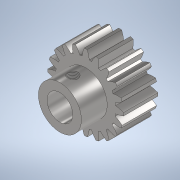
# Autodesk Inventor part: Spur Gear1
Saved by Autodesk Inventor 2020 (Build 240168000, 168)
## iProperties
CustomPartVersion: 1
Created: 2020-05-17
Part Number: Spur Gear1
Material: Steel, Mild
Document SubType Name: Modeling
Designer: Hesekiel
Categories: <?xml version="1.0" encoding="UTF-16"?> <MemberInstance><Categories><FamilyTemplate><FamilyTemplateParameter ValueType="xs:double" Id="1" ObjectReferenceKey="da_z" ObjectType="kUserParameterObject"/><FamilyTemplateParameter ValueType="xs:double" Id="2" ObjectReferenceKey="da_b" ObjectType="kUserParameterObject"/><FamilyTemplateParameter ValueType="xs:double" Id="3" ObjectReferenceKey="da_beta" ObjectType="kUserParameterObject"/><FamilyTemplateParameter ValueType="xs:double" Id="4" ObjectReferenceKey="da_da" ObjectType="kUserParameterObject"/><FamilyTemplateParameter ValueType="xs:double" Id="5" ObjectReferenceKey="da_aw" ObjectType="kUserParameterObject"/><FamilyTemplateParameter ValueType="xs:string" Id="6" ObjectReferenceKey="EAIAABAAAACIAQAAAAAAAIAAAAAAAAAA" ObjectType="83910656" SubObjectId="SurfaceGeometry"/></FamilyTemplate><ParamToTemplateMap><ParamToTemplate CategoryParameter="//CategoryParameter[@InternalName='046C89C9-8512-4d59-83FE-43B91F4F132A']" TemplateParameter="1"/><ParamToTemplate CategoryParameter="//CategoryParameter[@InternalName='2552DF32-E462-4b46-AEBF-C6C7768E72AC']" TemplateParameter="2"/><ParamToTemplate CategoryParameter="//CategoryParameter[@InternalName='C9EE641D-15FC-4fae-A226-E94C4372FDD7']" TemplateParameter="3"/><ParamToTemplate><ParamToTemplate CategoryParameter="//CategoryParameter[@InternalName='00B6519A-459B-49c7-AD84-2E56D39A5744']" ConstantValue="0.000000"/></ParamToTemplate><ParamToTemplate><ParamToTemplate CategoryParameter="//CategoryParameter[@InternalName='04B31F0E-C7A6-4894-AA32-9629BEFACF47']" ConstantValue="1.000000"/></ParamToTemplate><ParamToTemplate><ParamToTemplate CategoryParameter="//CategoryParameter[@InternalName='43CBEC2E-7847-49e7-A936-2F7889FCB2D9']" ConstantValue="0.250000"/></ParamToTemplate><ParamToTemplate><ParamToTemplate CategoryParameter="//CategoryParameter[@InternalName='B1EFC894-105D-4ebd-86BF-FA20ED196853']" ConstantValue="0.350000"/></ParamToTemplate><ParamToTemplate><ParamToTemplate CategoryParameter="//CategoryParameter[@InternalName='51175063-3D10-4879-93E8-6246FE8B403D']" ConstantValue="2060000000.000000"/></ParamToTemplate><ParamToTemplate><ParamToTemplate CategoryParameter="//CategoryParameter[@InternalName='A3A52E27-4454-46a9-B0BD-C932399B70AF']" ConstantValue="0.300000"/></ParamToTemplate><ParamToTemplate><ParamToTemplate CategoryParameter="//CategoryParameter[@InternalName='91B76062-C214-41d9-B1B9-14D2AB99603D']" ConstantValue="0.200000"/></ParamToTemplate><ParamToTemplate><ParamToTemplate CategoryParameter="//CategoryParameter[@InternalName='374E806E-8B8A-4dda-A9AA-1039D6500AD2']" ConstantValue="5.000000"/></ParamToTemplate><ParamToTemplate><ParamToTemplate CategoryParameter="//CategoryParameter[@InternalName='2D373A89-B862-43d6-8D0B-0CBF12AB9F6C']" ConstantValue="0.349066"/></ParamToTemplate><ParamToTemplate CategoryParameter="//CategoryParameter[@InternalName='37777632-D6A2-4fac-9D53-DB8ACD95C989']" TemplateParameter="4"/><ParamToTemplate CategoryParameter="//CategoryParameter[@InternalName='FD1017F1-B727-4f7e-9707-0F86F1FF9423']" TemplateParameter="5"/><ParamToTemplate><ParamToTemplate CategoryParameter="//CategoryParameter[@InternalName='9E1B4470-B2D3-4ff1-B813-535BB4CDF51A']" ConstantValue="3520000.000000"/></ParamToTemplate><ParamToTemplate><ParamToTemplate CategoryParameter="//CategoryParameter[@InternalName='F8452263-BFF6-458c-9FB1-07C4B99E95CD']" ConstantValue="11400000.000000"/></ParamToTemplate><ParamToTemplate><ParamToTemplate CategoryParameter="//CategoryParameter[@InternalName='3E3BB259-FD49-497f-8171-6EBC954A3479']" ConstantValue="2.000000"/></ParamToTemplate><ParamToTemplate CategoryParameter="//CategoryParameter[@InternalName='27C3BAF2-7550-4e4b-AE2C-0DB134B7D9B7']" TemplateParameter="6"/></ParamToTemplateMap><Category DisplayName="Gear" InternalName="DC85795E-93AB-48d5-8EEE-5A27447B64BD" Mnemonic="Gear"><CategoryParameter DisplayName="z" InternalName="046C89C9-8512-4d59-83FE-43B91F4F132A" Mnemonic="z"/><CategoryParameter DisplayName="b" InternalName="2552DF32-E462-4b46-AEBF-C6C7768E72AC" Mnemonic="b"/><CategoryParameter DisplayName="||b|" InternalName="C9EE641D-15FC-4fae-A226-E94C4372FDD7" Mnemonic="beta"/><CategoryParameter DisplayName="x" InternalName="00B6519A-459B-49c7-AD84-2E56D39A5744" Mnemonic="x"/><CategoryParameter DisplayName="a*" InternalName="04B31F0E-C7A6-4894-AA32-9629BEFACF47" Mnemonic="a"/><CategoryParameter DisplayName="c*" InternalName="43CBEC2E-7847-49e7-A936-2F7889FCB2D9" Mnemonic="c"/><CategoryParameter DisplayName="r|.f|*" InternalName="B1EFC894-105D-4ebd-86BF-FA20ED196853" Mnemonic="rf"/><CategoryParameter DisplayName="E" InternalName="51175063-3D10-4879-93E8-6246FE8B403D" Mnemonic="E"/><CategoryParameter DisplayName="||m|" InternalName="A3A52E27-4454-46a9-B0BD-C932399B70AF" Mnemonic="mi"/><Category DisplayName="SpurGear" InternalName="26C5A22E-A91E-4dfd-A3B3-23CCAFAE1764" Mnemonic="SpurGear"><CategoryParameter DisplayName="m" InternalName="91B76062-C214-41d9-B1B9-14D2AB99603D" Mnemonic="m"/><CategoryParameter DisplayName="P" InternalName="374E806E-8B8A-4dda-A9AA-1039D6500AD2" Mnemonic="PP"/><CategoryParameter DisplayName="||a|" InternalName="2D373A89-B862-43d6-8D0B-0CBF12AB9F6C" Mnemonic="alpha"/><CategoryParameter DisplayName="d|.a|" InternalName="37777632-D6A2-4fac-9D53-DB8ACD95C989" Mnemonic="da"/><CategoryParameter DisplayName="a|.w|" InternalName="FD1017F1-B727-4f7e-9707-0F86F1FF9423" Mnemonic="aw"/><CategoryParameter DisplayName="||s||.Flim|" InternalName="9E1B4470-B2D3-4ff1-B813-535BB4CDF51A" Mnemonic="sFlim"/><CategoryParameter DisplayName="||s||.Hlim|" InternalName="F8452263-BFF6-458c-9FB1-07C4B99E95CD" Mnemonic="sHlim"/><CategoryParameter DisplayName="type" InternalName="3E3BB259-FD49-497f-8171-6EBC954A3479" Mnemonic="type"/><CategoryParameter DisplayName="PitchDiameter" InternalName="27C3BAF2-7550-4e4b-AE2C-0DB134B7D9B7" Mnemonic="IDS_PITCHDIAM"/></Category></Category></Categories></MemberInstance>
Density: 7.85 g/cm^3
Appearance: Semi-Polished
Mass: 203.835 g
Surface Area: 100.654 cm^2
Volume: 25.9662 cm^3
Author: Hesekiel
Autodesk Inventor part; units mm, degrees
sketch "Sketch1" plane through (0, 0, 0) normal (0, 0, 1) x (1, 0, 0)
  circle A0 centre (0, 0) radius 22
  dimension "d0" = 44
  constraints: 1 centre point
  measures "d0" diameter of A0
extrude "Extrusion1" add sketch "Sketch1" along normal blind 20
ref_plane "Work Plane2" through (0, 0, 10) normal (0, 0, 1) x (1, 0, 0)
sketch "Sketch2" plane through (0, 0, 0) normal (0, 0, -1) x (-1, 0, 0)
  circle A0 centre (0, 0) radius 22 projected
  circle A1 centre (0, 0) radius 20
  dimension "d3" = 40
  constraints: 1 centre point, 1 coincident
  measures "d3" diameter of A1
surface extrude "Pitch Diameter" sketch "Sketch2" against normal through all shown no curves A1
ref_plane "Work Plane8" through (0, 0, 0) normal (0.9876883, 0.1564345, 0) x (0, 0, 1)
ref_plane "Work Plane9" through (0, 0, 0) normal (1, 0, 0) x (0, 1, 0)
spur gear teeth "Spur Gear" teeth 20 pitch diameter 40 tip diameter 44 root diameter 35 face width 20 start plane through (0, 0, 0) normal (0, 0, -1) x (-1, 0, 0)
sketch "Sketch3" plane through (0, 0, 20) normal (0, 0, 1) x (1, 0, 0)
  circle A0 centre (0, 0) radius 7.5
  dimension "d49" = 15
  constraints: 1 centre point, 1 coincident
  measures "d49" diameter of A0
extrude "Extrusion2" cut sketch "Sketch3" against normal up to surface (20 mm away)
sketch "Sketch4" plane through (0, 0, 20) normal (0, 0, 1) x (1, 0, 0)
  circle A0 centre (0, 0) radius 12.5
  circle A1 centre (0, 0) radius 7.5 projected
  arc A2 (-7.6146, 20.6402) -> (-7.3265, 15.8925) centre (8.9064, 19.2599) ccw projected
  arc A3 (-7.3265, 15.8925) -> (-8.5509, 15.2687) centre (0, 0) ccw projected
  arc A4 (-8.5509, 15.2687) -> (-12.2225, 18.2923) centre (-20.8166, 4.1153) ccw projected
  arc A5 (-12.2225, 18.2923) -> (-13.6201, 17.277) centre (0, 0) ccw projected
  arc A6 (-13.6201, 17.277) -> (-11.879, 12.8506) centre (2.5188, 21.0695) ccw projected
  arc A7 (-11.879, 12.8506) -> (-12.8506, 11.879) centre (0, 0) ccw projected
  arc A8 (-12.8506, 11.879) -> (-17.277, 13.6201) centre (-21.0695, -2.5188) ccw projected
  arc A9 (-17.277, 13.6201) -> (-18.2923, 12.2225) centre (0, 0) ccw projected
  arc A10 (-18.2923, 12.2225) -> (-15.2687, 8.5509) centre (-4.1153, 20.8166) ccw projected
  arc A11 (-15.2687, 8.5509) -> (-15.8925, 7.3265) centre (0, 0) ccw projected
  arc A12 (-15.8925, 7.3265) -> (-20.6402, 7.6146) centre (-19.2599, -8.9064) ccw projected
  arc A13 (-20.6402, 7.6146) -> (-21.174, 5.9717) centre (0, 0) ccw projected
  arc A14 (-21.174, 5.9717) -> (-17.1637, 3.4141) centre (-10.3466, 18.5261) ccw projected
  arc A15 (-17.1637, 3.4141) -> (-17.3787, 2.0569) centre (0, 0) ccw projected
  arc A16 (-17.3787, 2.0569) -> (-21.983, 0.8637) centre (-15.565, -14.4221) ccw projected
  arc A17 (-21.983, 0.8637) -> (-21.983, -0.8637) centre (0, 0) ccw projected
  arc A18 (-21.983, -0.8637) -> (-17.3787, -2.0569) centre (-15.565, 14.4221) ccw projected
  arc A19 (-17.3787, -2.0569) -> (-17.1637, -3.4141) centre (0, 0) ccw projected
  arc A20 (-17.1637, -3.4141) -> (-21.174, -5.9717) centre (-10.3466, -18.5261) ccw projected
  arc A21 (-21.174, -5.9717) -> (-20.6402, -7.6146) centre (0, 0) ccw projected
  arc A22 (-20.6402, -7.6146) -> (-15.8925, -7.3265) centre (-19.2599, 8.9064) ccw projected
  arc A23 (-15.8925, -7.3265) -> (-15.2687, -8.5509) centre (0, 0) ccw projected
  arc A24 (-15.2687, -8.5509) -> (-18.2923, -12.2225) centre (-4.1153, -20.8166) ccw projected
  arc A25 (-18.2923, -12.2225) -> (-17.277, -13.6201) centre (0, 0) ccw projected
  arc A26 (-17.277, -13.6201) -> (-12.8506, -11.879) centre (-21.0695, 2.5188) ccw projected
  arc A27 (-12.8506, -11.879) -> (-11.879, -12.8506) centre (0, 0) ccw projected
  arc A28 (-11.879, -12.8506) -> (-13.6201, -17.277) centre (2.5188, -21.0695) ccw projected
  arc A29 (-13.6201, -17.277) -> (-12.2225, -18.2923) centre (0, 0) ccw projected
  arc A30 (-12.2225, -18.2923) -> (-8.5509, -15.2687) centre (-20.8166, -4.1153) ccw projected
  arc A31 (-8.5509, -15.2687) -> (-7.3265, -15.8925) centre (0, 0) ccw projected
  arc A32 (-7.3265, -15.8925) -> (-7.6146, -20.6402) centre (8.9064, -19.2599) ccw projected
  arc A33 (-7.6146, -20.6402) -> (-5.9717, -21.174) centre (0, 0) ccw projected
  arc A34 (-5.9717, -21.174) -> (-3.4141, -17.1637) centre (-18.5261, -10.3466) ccw projected
  arc A35 (-3.4141, -17.1637) -> (-2.0569, -17.3787) centre (0, 0) ccw projected
  arc A36 (-2.0569, -17.3787) -> (-0.8637, -21.983) centre (14.4221, -15.565) ccw projected
  arc A37 (-0.8637, -21.983) -> (0.8637, -21.983) centre (0, 0) ccw projected
  arc A38 (0.8637, -21.983) -> (2.0569, -17.3787) centre (-14.4221, -15.565) ccw projected
  arc A39 (2.0569, -17.3787) -> (3.4141, -17.1637) centre (0, 0) ccw projected
  arc A40 (3.4141, -17.1637) -> (5.9717, -21.174) centre (18.5261, -10.3466) ccw projected
  arc A41 (5.9717, -21.174) -> (7.6146, -20.6402) centre (0, 0) ccw projected
  arc A42 (7.6146, -20.6402) -> (7.3265, -15.8925) centre (-8.9064, -19.2599) ccw projected
  arc A43 (7.3265, -15.8925) -> (8.5509, -15.2687) centre (0, 0) ccw projected
  arc A44 (8.5509, -15.2687) -> (12.2225, -18.2923) centre (20.8166, -4.1153) ccw projected
  arc A45 (12.2225, -18.2923) -> (13.6201, -17.277) centre (0, 0) ccw projected
  arc A46 (13.6201, -17.277) -> (11.879, -12.8506) centre (-2.5188, -21.0695) ccw projected
  arc A47 (11.879, -12.8506) -> (12.8506, -11.879) centre (0, 0) ccw projected
  arc A48 (12.8506, -11.879) -> (17.277, -13.6201) centre (21.0695, 2.5188) ccw projected
  arc A49 (17.277, -13.6201) -> (18.2923, -12.2225) centre (0, 0) ccw projected
  arc A50 (18.2923, -12.2225) -> (15.2687, -8.5509) centre (4.1153, -20.8166) ccw projected
  arc A51 (15.2687, -8.5509) -> (15.8925, -7.3265) centre (0, 0) ccw projected
  arc A52 (15.8925, -7.3265) -> (20.6402, -7.6146) centre (19.2599, 8.9064) ccw projected
  arc A53 (20.6402, -7.6146) -> (21.174, -5.9717) centre (0, 0) ccw projected
  arc A54 (21.174, -5.9717) -> (17.1637, -3.4141) centre (10.3466, -18.5261) ccw projected
  arc A55 (17.1637, -3.4141) -> (17.3787, -2.0569) centre (0, 0) ccw projected
  arc A56 (17.3787, -2.0569) -> (21.983, -0.8637) centre (15.565, 14.4221) ccw projected
  arc A57 (21.983, -0.8637) -> (21.983, 0.8637) centre (0, 0) ccw projected
  arc A58 (21.983, 0.8637) -> (17.3787, 2.0569) centre (15.565, -14.4221) ccw projected
  arc A59 (17.3787, 2.0569) -> (17.1637, 3.4141) centre (0, 0) ccw projected
  arc A60 (17.1637, 3.4141) -> (21.174, 5.9717) centre (10.3466, 18.5261) ccw projected
  arc A61 (21.174, 5.9717) -> (20.6402, 7.6146) centre (0, 0) ccw projected
  arc A62 (20.6402, 7.6146) -> (15.8925, 7.3265) centre (19.2599, -8.9064) ccw projected
  arc A63 (15.8925, 7.3265) -> (15.2687, 8.5509) centre (0, 0) ccw projected
  arc A64 (15.2687, 8.5509) -> (18.2923, 12.2225) centre (4.1153, 20.8166) ccw projected
  arc A65 (18.2923, 12.2225) -> (17.277, 13.6201) centre (0, 0) ccw projected
  arc A66 (17.277, 13.6201) -> (12.8506, 11.879) centre (21.0695, -2.5188) ccw projected
  arc A67 (12.8506, 11.879) -> (11.879, 12.8506) centre (0, 0) ccw projected
  arc A68 (11.879, 12.8506) -> (13.6201, 17.277) centre (-2.5188, 21.0695) ccw projected
  arc A69 (13.6201, 17.277) -> (12.2225, 18.2923) centre (0, 0) ccw projected
  arc A70 (12.2225, 18.2923) -> (8.5509, 15.2687) centre (20.8166, 4.1153) ccw projected
  arc A71 (8.5509, 15.2687) -> (7.3265, 15.8925) centre (0, 0) ccw projected
  arc A72 (7.3265, 15.8925) -> (7.6146, 20.6402) centre (-8.9064, 19.2599) ccw projected
  arc A73 (7.6146, 20.6402) -> (5.9717, 21.174) centre (0, 0) ccw projected
  arc A74 (5.9717, 21.174) -> (3.4141, 17.1637) centre (18.5261, 10.3466) ccw projected
  arc A75 (3.4141, 17.1637) -> (2.0569, 17.3787) centre (0, 0) ccw projected
  arc A76 (2.0569, 17.3787) -> (0.8637, 21.983) centre (-14.4221, 15.565) ccw projected
  arc A77 (0.8637, 21.983) -> (-0.8637, 21.983) centre (0, 0) ccw projected
  arc A78 (-0.8637, 21.983) -> (-2.0569, 17.3787) centre (14.4221, 15.565) ccw projected
  arc A79 (-2.0569, 17.3787) -> (-3.4141, 17.1637) centre (0, 0) ccw projected
  arc A80 (-3.4141, 17.1637) -> (-5.9717, 21.174) centre (-18.5261, 10.3466) ccw projected
  arc A81 (-5.9717, 21.174) -> (-7.6146, 20.6402) centre (0, 0) ccw projected
  dimension "d52" = 25
  constraints: 1 centre point, 1 coincident
  measures "d52" diameter of A0
extrude "Extrusion4" add sketch "Sketch4" along normal blind 15 contours A0
ref_plane "Work Plane11" through (0, 12.5, 20) normal (0, 1, 0) x (-1, 0, 0)
sketch "Sketch5" plane through (0, 12.5, 20) normal (0, 1, 0) x (-1, 0, 0)
  line L0 (12.5, 15) -> (-12.5, 15) projected
  line L1 (-12.5, 0) -> (12.5, 0) projected
  line L2 (-7.5, 15) -> (7.5, 15) projected
  line L3 (0, 15) -> (0, 0)
  line L4 (-0.8637, 0) -> (0.8637, 0) projected
  circle A0 centre (0, 7.5) radius 3
  point P0 (0, -20)
  dimension "d57" = 6
  constraints: 3 midpoint, 2 end point, 1 centre point
  measures "d57" diameter of A0
extrude "Extrusion5" cut sketch "Sketch5" against normal up to surface
thread "Thread1" size "M6x0.75" class "6H" standard "ANSI Metric M Profile" full length
equation "\"d0\" = da_da"
equation "\"d1\" = da_b"
equation "\"d3\" = da_dw"
equation "\"da_da\" = 44"
equation "\"da_b\" = 20"
equation "\"da_dw\" = 40"
body "Solid1"
body "Srf1"
